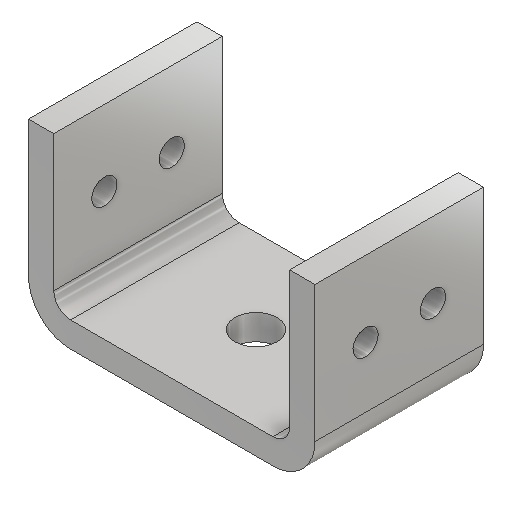
# Autodesk Inventor part: LCBN_ALU_3mm_Y_Axis_Idler_Stiffener_Top
Saved by Autodesk Inventor 2026.1 (Build 301233000, 233)
## iProperties
Created: 2017-05-25
Part Number: LCBN_ALU_3mm_Y_Axis_Idler_Stiffener_Top
Material: Ogólny
Document SubType Name: Modeling
Designer: Andrzej
Density: 1 g/cm^3
Appearance: Aluminium - ciemne
Mass: 3.89353 g
Surface Area: 32.7963 cm^2
Volume: 3.89353 cm^3
Author: Andrzej
Autodesk Inventor part; units mm, degrees
ref_plane "YZ Plane" through (0, 0, 0) normal (1, 0, 0) x (0, 1, 0)
ref_plane "XZ Plane" through (0, 0, 0) normal (0, 1, 0) x (-1, 0, 0)
ref_plane "XY Plane" through (0, 0, 0) normal (0, 0, 1) x (1, 0, 0)
sketch "Szkic1" plane through (0, 0, 0) normal (0, 0, 1) x (1, 0, 0)
  line L0 (-12.5286, 12.4626) -> (59.4714, 12.4626)
  line L1 (59.4714, 12.4626) -> (59.4714, -7.5374)
  line L2 (59.4714, -7.5374) -> (-12.5286, -7.5374)
  line L3 (-12.5286, -7.5374) -> (-12.5286, 12.4626)
  line L4 (11.4714, 12.4626) -> (11.4714, -7.5374)
  line L5 (35.4714, 12.4626) -> (35.4714, -7.5374)
  point P0 (0, 0)
  dimension "d0" = 72
  dimension "d1" = 20
  dimension "d5" = 24
  dimension "d6" = 24
  constraints: 12 end point, 4 point on line, 3 perpendicular, 2 parallel, 1 horizontal
  measures "d0" distance of L1.end L2.end
  measures "d1" distance of L2.end L0.start
  measures "d5" distance between parallel lines of L3 L4
  measures "d6" distance between parallel lines of L1 L5
extrude "Wyciągnięcie proste1" add sketch "Szkic1" along normal blind 3
bend part "Gięcie części1" radius 5 angle 90 line through (11.4714, 12.4626, 0) along (0, -1, 0) centre toward (0, 0, 1) moving side (-1, 0, 0) both sides no
bend part "Gięcie części2" radius 5 angle 90 line through (35.4714, 12.4626, 0) along (0, -1, 0) centre toward (0, 0, 1) moving side (1, 0, 0) both sides no
sketch "Szkic2" plane through (0, 0, 0) normal (0, 0, -1) x (-1, 0, 0)
  line L0 (-35.4714, -7.5374) -> (-35.4714, 12.4626) projected
  line L1 (-35.4714, -7.5374) -> (-11.4714, -7.5374) projected
  line L2 (-11.4714, 12.4626) -> (-11.4714, -7.5374) projected
  line L3 (-11.4714, 12.4626) -> (-35.4714, 12.4626) projected
  point P0 (0, 0)
  point P1 (-23.4714, 2.4626)
  dimension "d11" = 10
  dimension "d12" = 12
  dimension "d13" = 24
  measures "d11" distance from line of L3 point (-23.471, 2.463)
  measures "d12" distance from line of L2 point (-23.471, 2.463)
  measures "d13" distance of L0.start L1.end
hole "Otwór1" at (23.4714, 2.4626, 0) direction (0, 0, 1) diameter 5 depth 8 tip angle 118
sketch "Szkic3" plane through (6.4714, -7.5374, 5) normal (-1, 0, 0) x (0, 0, 1)
  line L0 (0, 20) -> (0, 0) projected
  line L1 (0, 0) -> (16.146, 0) projected
  line L2 (16.146, 0) -> (16.146, 20) projected
  line L3 (16.146, 20) -> (0, 20) projected
  line L4 (20.2, 0) -> (20.2, 20)
  line L5 (0, 20) -> (0, 0) projected
  line L6 (0, 20) -> (-5, 20) projected
  line L7 (-5, 20) -> (-5, 0) projected
  line L8 (-5, 0) -> (0, 0) projected
  point P0 (-5, 7.5374)
  point P1 (7.2, 6)
  point P2 (7.2, 14)
  dimension "d21" = 6
  dimension "d22" = 6
  dimension "d25" = 13
  dimension "d27" = 13
  dimension "d28" = 25.2
  constraints: 2 end point, 1 vertical
  measures "d21" distance from line of L1 point (7.2, 6)
  measures "d22" distance from line of L3 point (7.2, 14)
  measures "d25" distance from line of point (7.2, 6) L4
  measures "d27" distance from line of L4 point (7.2, 14)
  measures "d28" distance between parallel lines of L7 L4
hole "Otwór2" at (6.4714, -1.5374, 12.2) at (6.4714, 6.4626, 12.2) direction (1, 0, 0) diameter 3 end through all
equation "\"d5\" = d6"
equation "\"d22\" = d21"
equation "\"d27\" = d25"
